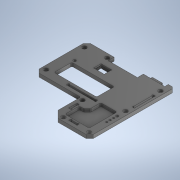
# Autodesk Inventor part: Cockpit_side_frame
Saved by Autodesk Inventor 2022.3 (Build 263350000, 350)
## iProperties
Part Number: Cockpit_side_frame
Material: アセタール樹脂、黒
Document SubType Name: Modeling
Designer: Masato Kubotera
Density: 1.425 g/cm^3
Appearance: 滑らか - 黒
Description: POM T5
Mass: 49.7941 g
Surface Area: 232.095 cm^2
Volume: 34.9432 cm^3
Author: Masato Kubotera
Autodesk Inventor part; units mm, degrees
ref_plane "YZ Plane" through (0, 0, 0) normal (1, 0, 0) x (0, 1, 0)
ref_plane "XZ Plane" through (0, 0, 0) normal (0, 1, 0) x (-1, 0, 0)
ref_plane "XY Plane" through (0, 0, 0) normal (0, 0, 1) x (1, 0, 0)
derived "Trunk_basis.ipt"
sketch "スケッチ1" plane through (0, 0, 0) normal (0, 1, 0) x (-1, 0, 0)
  line L0 (0, 22) -> (0, -142.9) construction
  circle A0 centre (5, 0) radius 10.5 construction
  line L1 (-7, 16) -> (36, 16) construction
  line L2 (36, 16) -> (36, -16) construction
  line L3 (36, -16) -> (-7, -16) construction
  line L4 (-7, -16) -> (-7, 16) construction
  line L5 (-7, 16) -> (36, -16) construction
  line L6 (36, 16) -> (-7, -16) construction
  line L7 (33, 13.5) -> (6, 13.5) construction
  line L8 (6, 13.5) -> (6, -13.5) construction
  line L9 (6, -13.5) -> (33, -13.5) construction
  line L10 (33, -13.5) -> (33, 13.5) construction
  line L11 (33, 13.5) -> (6, -13.5) construction
  line L12 (6, 13.5) -> (33, -13.5) construction
  line L13 (-7, 0) -> (36, 0) construction
  arc A1 (5, 16) -> (-7, 10.583) centre (5, 0) ccw construction
  line L14 (43.75, -16.25) -> (5, -16.25)
  line L15 (5, 16.25) -> (43.75, 16.25)
  line L16 (44.75, 15.25) -> (44.75, -15.25)
  arc A2 (5, 16.25) -> (-6.7376, 11.2379) centre (5, 0) ccw
  arc A3 (-6.7376, 11.2379) -> (-7.25, 9.9174) centre (-6.2711, 10.2972) ccw
  circle A4 centre (6, 13.5) radius 1.35
  line L17 (19.5, 13.5) -> (19.5, -13.5) construction
  circle A5 centre (33, 13.5) radius 1.35
  line L18 (-15, 22) -> (-20, 17)
  line L19 (-20, 17) -> (-20, -19)
  line L20 (-20, -19) -> (-28.5, -27.5)
  line L21 (-28.5, -27.5) -> (-28.5, -103)
  line L22 (57.5, -22.5) -> (57.5, 17)
  line L23 (57.5, 17) -> (52.5, 22)
  line L24 (52.5, 22) -> (-15, 22)
  line L25 (-35.5597, -116.5529) -> (-28.5, -142.9)
  line L26 (-16, -139) -> (-16, -94) construction
  line L27 (-7.5, -140.4849) -> (-7.5, -142.9)
  line L28 (-7.5, -142.9) -> (7.5, -142.9)
  line L29 (7.5, -140.4849) -> (7.5, -142.9)
  arc A6 (-7.5, -140.4849) -> (-8.9849, -139) centre (-8.2425, -139.7425) ccw
  line L30 (-17.5, -138.9955) -> (-17.5, -133) construction
  line L31 (-19, -133) -> (-16, -133) construction
  line L32 (-19, -133) -> (-19, -139) construction
  line L33 (-16, -133) -> (-16, -139) construction
  line L34 (-15, 22) -> (-10, 22) construction
  line L35 (-10, 22) -> (-10, -22) construction
  line L36 (-10, -22) -> (-15, -22) construction
  line L37 (-15, -22) -> (-15, 22) construction
  line L38 (-15, 22) -> (-10, -22) construction
  line L39 (-10, 22) -> (-15, -22) construction
  line L40 (-12.5, 22) -> (-12.5, -22) construction
  line L41 (-10, 0) -> (-15, 0) construction
  circle A7 centre (-12.5, 17.75) radius 1.6
  line L42 (-15, 10) -> (-12.5, 10) construction
  line L43 (-12.5, 10) -> (-12.5, -10) construction
  line L44 (-12.5, -10) -> (-15, -10) construction
  line L45 (-15, -10) -> (-15, 10) construction
  line L46 (-15, 10) -> (-12.5, -10) construction
  line L47 (-12.5, 10) -> (-15, -10) construction
  line L48 (-12.25, 10.25) -> (-15.25, 10.25)
  line L49 (-15.25, 8.15) -> (-15.25, -8.15)
  line L50 (-15.25, -10.25) -> (-12.25, -10.25)
  line L51 (-12.25, -8.15) -> (-12.25, 8.15)
  line L52 (-12.25, 10.25) -> (-15.25, -10.25) construction
  line L53 (-15.25, 10.25) -> (-12.25, -10.25) construction
  arc A8 (-15.25, 10.25) -> (-15.25, 8.15) centre (-15.25, 9.2) ccw
  line L54 (-13.75, 10) -> (-13.75, -10) construction
  arc A9 (-12.25, 8.15) -> (-12.25, 10.25) centre (-12.25, 9.2) ccw
  circle A10 centre (-12.5, -17.75) radius 1.6
  arc A11 (-15.25, -8.15) -> (-15.25, -10.25) centre (-15.25, -9.2) ccw
  arc A12 (-12.25, -10.25) -> (-12.25, -8.15) centre (-12.25, -9.2) ccw
  line L55 (36, 14.4) -> (44.5, 14.4) construction
  line L56 (44.5, 14.4) -> (44.5, -14.4) construction
  line L57 (36, -14.4) -> (44.5, -14.4) construction
  line L58 (49.95, 7.95) -> (49.95, -7.95)
  line L59 (52.5, 0) -> (47.5, 0) construction
  line L60 (47.5, 22) -> (52.5, 22) construction
  line L61 (52.55, -7.95) -> (52.55, 7.95)
  line L62 (51.25, 10) -> (51.25, -10) construction
  line L63 (52.5, 10) -> (50, -10) construction
  line L64 (52.5, -10) -> (50, -10) construction
  line L65 (52.5, 10) -> (52.5, -10) construction
  line L66 (50, 10) -> (52.5, -10) construction
  line L67 (49.95, -10.05) -> (52.55, -10.05)
  line L68 (49.95, 10.05) -> (52.55, -10.05) construction
  line L69 (52.55, 10.05) -> (49.95, -10.05) construction
  line L70 (52.5, -22) -> (47.5, -22) construction
  line L71 (47.5, 22) -> (52.5, -22) construction
  line L72 (52.5, 22) -> (52.5, -22) construction
  line L73 (52.5, 22) -> (47.5, -22) construction
  line L74 (50, 22) -> (50, -22) construction
  line L75 (47.5, -22) -> (47.5, 22) construction
  circle A13 centre (50, -17.75) radius 1.6
  arc A14 (52.55, -10.05) -> (52.55, -7.95) centre (52.55, -9) ccw
  line L76 (50, -10) -> (50, 10) construction
  arc A15 (49.95, -7.95) -> (49.95, -10.05) centre (49.95, -9) ccw
  arc A16 (49.95, 10.05) -> (49.95, 7.95) centre (49.95, 9) ccw
  arc A17 (52.55, 7.95) -> (52.55, 10.05) centre (52.55, 9) ccw
  line L77 (50, 10) -> (52.5, 10) construction
  line L78 (52.55, 10.05) -> (49.95, 10.05)
  circle A18 centre (50, 17.75) radius 1.6
  circle A19 centre (5, 0) radius 16 construction
  arc A20 (-6.7376, -11.2379) -> (5, -16.25) centre (5, 0) ccw
  arc A21 (-7.25, -9.9174) -> (-6.7376, -11.2379) centre (-6.2711, -10.2972) ccw
  line L79 (-7.25, -9.9174) -> (-7.25, 9.9174)
  line L80 (17.5, -138.9955) -> (17.5, -133) construction
  line L81 (19, -133) -> (19, -139) construction
  line L82 (16, -133) -> (16, -139) construction
  line L83 (19, -133) -> (16, -133) construction
  circle A22 centre (6, -13.5) radius 1.35
  circle A23 centre (33, -13.5) radius 1.35
  line L84 (-25.5, -142.9) -> (-7.5, -142.9) construction
  line L85 (25.5, -142.9) -> (7.5, -142.9) construction
  line L86 (-23.5, -22.5) -> (57.5, -22.5) construction
  line L87 (57.5, -22.5) -> (57.5, -103)
  circle A24 centre (-13.5, -55) radius 1.75
  line L88 (-11.5, -59) -> (45.5, -59)
  line L89 (47.5, -61) -> (47.5, -82.5)
  line L90 (45.5, -84.5) -> (-11.5, -84.5)
  line L91 (-13.5, -82.5) -> (-13.5, -61)
  line L92 (-13.5, -59) -> (47.5, -84.5) construction
  line L93 (47.5, -59) -> (-13.5, -84.5) construction
  line L94 (-11.5, -27.5) -> (45.5, -27.5)
  line L95 (47.5, -29.5) -> (47.5, -49)
  line L96 (45.5, -51) -> (-11.5, -51)
  line L97 (-13.5, -49) -> (-13.5, -29.5)
  line L98 (-13.5, -27.5) -> (47.5, -51) construction
  line L99 (47.5, -27.5) -> (-13.5, -51) construction
  line L100 (-23.5, -108) -> (-28.5, -103)
  circle A25 centre (-20.5415, -102) radius 1.6
  line L101 (-25.7227, -96) -> (25.7227, -96)
  line L102 (25.7227, -96) -> (34.9603, -112)
  line L103 (35.5597, -116.5529) -> (28.5, -142.9)
  line L104 (-25.7227, -96) -> (-34.9603, -112)
  line L105 (57.5, -103) -> (52.5, -108)
  arc A26 (-11.5, -27.5) -> (-13.5, -29.5) centre (-11.5, -29.5) ccw
  arc A27 (-13.5, -49) -> (-11.5, -51) centre (-11.5, -49) ccw
  arc A28 (45.5, -51) -> (47.5, -49) centre (45.5, -49) ccw
  arc A29 (47.5, -29.5) -> (45.5, -27.5) centre (45.5, -29.5) ccw
  arc A30 (-11.5, -59) -> (-13.5, -61) centre (-11.5, -61) ccw
  arc A31 (-13.5, -82.5) -> (-11.5, -84.5) centre (-11.5, -82.5) ccw
  arc A32 (45.5, -84.5) -> (47.5, -82.5) centre (45.5, -82.5) ccw
  arc A33 (47.5, -61) -> (45.5, -59) centre (45.5, -61) ccw
  line L106 (-23.5, -108) -> (52.5, -108)
  line L107 (-25.5, -139) -> (-25.5, -142.9)
  line L108 (-25.5, -142.9) -> (-28.5, -142.9)
  line L109 (-17.9813, -99.3843) -> (-16.9961, -101.0907)
  line L110 (-16.9961, -102.9093) -> (-17.9813, -104.6157)
  line L111 (-19.5563, -105.525) -> (-21.5266, -105.525)
  line L112 (-23.1016, -104.6157) -> (-24.0868, -102.9093)
  line L113 (-24.0868, -101.0907) -> (-23.1016, -99.3843)
  line L114 (-21.5266, -98.475) -> (-19.5563, -98.475)
  line L115 (-16, -94) -> (16, -94) construction
  arc A34 (-24.0868, -101.0907) -> (-24.0868, -102.9093) centre (-23.5618, -102) ccw
  arc A35 (-23.1016, -104.6157) -> (-21.5266, -105.525) centre (-22.0516, -104.6157) ccw
  arc A36 (-19.5563, -105.525) -> (-17.9813, -104.6157) centre (-19.0313, -104.6157) ccw
  arc A37 (-16.9961, -102.9093) -> (-16.9961, -101.0907) centre (-17.5211, -102) ccw
  arc A38 (-17.9813, -99.3843) -> (-19.5563, -98.475) centre (-19.0313, -99.3843) ccw
  arc A39 (-21.5266, -98.475) -> (-23.1016, -99.3843) centre (-22.0516, -99.3843) ccw
  line L116 (16, -139) -> (16, -94) construction
  line L117 (16, -94) -> (-16, -94) construction
  line L118 (-25.5, -139) -> (-8.9849, -139)
  line L119 (25.5, -142.9) -> (28.5, -142.9)
  arc A40 (8.9849, -139) -> (7.5, -140.4849) centre (8.2425, -139.7425) ccw
  circle A41 centre (29.7641, -115) radius 1.25
  line L120 (33.4891, -124.2803) -> (21.898, -121.1745) construction
  line L121 (29.7641, -115) -> (25.623, -130.4548) construction
  circle A42 centre (29.7641, -115) radius 6 construction
  circle A43 centre (-20.5415, -102) radius 6 construction
  line L122 (1.9319, -109.4824) -> (7.5588, -130.4824)
  line L123 (5.6269, -133) -> (-5.6269, -133)
  line L124 (5.3151, -110.5176) -> (10.942, -131.5176)
  line L125 (12.8739, -133) -> (17.1947, -133)
  line L126 (19.1266, -131.5176) -> (24.7535, -110.5176)
  line L127 (22.8217, -108) -> (7.2469, -108)
  circle A44 centre (25.623, -130.4548) radius 1.25
  circle A45 centre (25.623, -130.4548) radius 6 construction
  line L128 (-1.9319, -109.4824) -> (-7.5588, -130.4824)
  arc A46 (1.9319, -109.4824) -> (-1.9319, -109.4824) centre (0, -110) ccw
  arc A47 (-7.5588, -130.4824) -> (-5.6269, -133) centre (-5.6269, -131) ccw
  arc A48 (5.6269, -133) -> (7.5588, -130.4824) centre (5.6269, -131) ccw
  arc A49 (7.2469, -108) -> (5.3151, -110.5176) centre (7.2469, -110) ccw
  arc A50 (24.7535, -110.5176) -> (22.8217, -108) centre (22.8217, -110) ccw
  arc A51 (17.1947, -133) -> (19.1266, -131.5176) centre (17.1947, -131) ccw
  arc A52 (10.942, -131.5176) -> (12.8739, -133) centre (12.8739, -131) ccw
  arc A53 (-5.3151, -110.5176) -> (-7.2469, -108) centre (-7.2469, -110) ccw
  line L129 (-22.8217, -108) -> (-7.2469, -108)
  line L130 (-5.3151, -110.5176) -> (-10.942, -131.5176)
  arc A54 (-22.8217, -108) -> (-24.7535, -110.5176) centre (-22.8217, -110) ccw
  line L131 (-19.1266, -131.5176) -> (-24.7535, -110.5176)
  arc A55 (-19.1266, -131.5176) -> (-17.1947, -133) centre (-17.1947, -131) ccw
  line L132 (-12.8739, -133) -> (-17.1947, -133)
  arc A56 (-12.8739, -133) -> (-10.942, -131.5176) centre (-12.8739, -131) ccw
  circle A57 centre (-29.7641, -115) radius 1.25
  circle A58 centre (-25.623, -130.4548) radius 1.25
  arc A59 (35.5597, -116.5529) -> (34.9603, -112) centre (29.7641, -115) ccw
  arc A60 (-34.9603, -112) -> (-35.5597, -116.5529) centre (-29.7641, -115) ccw
  arc A61 (-24.0151, -139) -> (-25.5, -140.4849) centre (-24.7575, -139.7425) ccw
  line L133 (25.5, -139) -> (25.5, -142.9)
  arc A62 (25.5, -140.4849) -> (24.0151, -139) centre (24.7575, -139.7425) ccw
  line L134 (25.5, -139) -> (8.9849, -139)
  line L135 (21.5266, -98.475) -> (19.5563, -98.475)
  line L136 (16.9961, -102.9093) -> (17.9813, -104.6157)
  arc A63 (21.5266, -105.525) -> (23.1016, -104.6157) centre (22.0516, -104.6157) ccw
  circle A64 centre (20.5415, -102) radius 1.6
  line L137 (24.0868, -101.0907) -> (23.1016, -99.3843)
  arc A65 (24.0868, -102.9093) -> (24.0868, -101.0907) centre (23.5618, -102) ccw
  line L138 (23.1016, -104.6157) -> (24.0868, -102.9093)
  arc A66 (23.1016, -99.3843) -> (21.5266, -98.475) centre (22.0516, -99.3843) ccw
  line L139 (19.5563, -105.525) -> (21.5266, -105.525)
  arc A67 (19.5563, -98.475) -> (17.9813, -99.3843) centre (19.0313, -99.3843) ccw
  arc A68 (17.9813, -104.6157) -> (19.5563, -105.525) centre (19.0313, -104.6157) ccw
  line L140 (17.9813, -99.3843) -> (16.9961, -101.0907)
  arc A69 (16.9961, -101.0907) -> (16.9961, -102.9093) centre (17.5211, -102) ccw
  line L141 (16, -139) -> (16, -94) construction
  circle A70 centre (20.5415, -102) radius 6 construction
  arc A71 (29.5045, -117.5445) -> (31.2612, -117.0738) centre (30.247, -116.802) ccw construction
  line L142 (31.8379, -116.4971) -> (31.2612, -117.0738) construction
  line L143 (29.5045, -117.5445) -> (28.7167, -117.3334) construction
  arc A72 (27.4307, -116.0474) -> (28.7167, -117.3334) centre (28.4449, -116.3192) ccw construction
  line L144 (27.4307, -116.0474) -> (27.2196, -115.2596) construction
  line L145 (27.6903, -113.5029) -> (28.267, -112.9262) construction
  arc A73 (30.0237, -112.4555) -> (28.267, -112.9262) centre (29.2813, -113.198) ccw construction
  arc A74 (27.6903, -113.5029) -> (27.2196, -115.2596) centre (27.9621, -114.5171) ccw construction
  line L146 (30.0237, -112.4555) -> (30.8116, -112.6666) construction
  arc A75 (31.8379, -116.4971) -> (32.3086, -114.7404) centre (31.5662, -115.4829) ccw construction
  arc A76 (32.0975, -113.9526) -> (30.8116, -112.6666) centre (31.0833, -113.6808) ccw construction
  line L147 (32.0975, -113.9526) -> (32.3086, -114.7404) construction
  line L148 (-20.5415, -102) -> (20.5415, -102) construction
  circle A77 centre (0, -102) radius 1.6
  line L149 (0.4078, -104.525) -> (-0.4078, -104.525)
  arc A78 (-0.4078, -99.475) -> (-1.9828, -100.3843) centre (-0.9328, -100.3843) ccw
  arc A79 (0.4078, -104.525) -> (1.9828, -103.6157) centre (0.9328, -103.6157) ccw
  line L150 (2.3906, -102.9093) -> (1.9828, -103.6157)
  line L151 (-0.4078, -99.475) -> (0.4078, -99.475)
  arc A80 (1.9828, -100.3843) -> (0.4078, -99.475) centre (0.9328, -100.3843) ccw
  line L152 (1.9828, -100.3843) -> (2.3906, -101.0907)
  arc A81 (2.3906, -102.9093) -> (2.3906, -101.0907) centre (1.8656, -102) ccw
  line L153 (-2.3906, -101.0907) -> (-1.9828, -100.3843)
  arc A82 (-2.3906, -101.0907) -> (-2.3906, -102.9093) centre (-1.8656, -102) ccw
  line L154 (-1.9828, -103.6157) -> (-2.3906, -102.9093)
  arc A83 (-1.9828, -103.6157) -> (-0.4078, -104.525) centre (-0.9328, -103.6157) ccw
  circle A84 centre (0, -102) radius 1.25
  arc A85 (44.75, 15.25) -> (43.75, 16.25) centre (43.75, 15.25) ccw
  arc A86 (43.75, -16.25) -> (44.75, -15.25) centre (43.75, -15.25) ccw
  circle A87 centre (-22.75, -31.75) radius 3
  circle A88 centre (-22.75, -86.75) radius 3
  line L155 (-23.5, -96) -> (-28.5, -91) construction
  line L156 (-26, -93.5) -> (-22.75, -93.5) construction
  line L157 (-26, -25) -> (-22.75, -25) construction
  line L158 (-26, -25) -> (-26, -93.5) construction
  line L159 (-22.75, -25) -> (-22.75, -93.5) construction
  line L160 (-22.75, -59.25) -> (-28.5, -59.25) construction
  point P0 (0, 0)
  point P1 (14.5, 0)
  point P2 (19.5, 0)
  point P3 (44.75, 16.25)
  point P4 (-7.25, 10.6771)
  point P5 (19.5, 0)
  point P6 (-12.5, 0)
  point P7 (-13.75, 0)
  point P8 (44.75, 14.4)
  point P9 (44.75, -14.4)
  point P10 (51.25, 0)
  point P11 (50, 0)
  point P12 (44.75, -16.25)
  point P13 (17, -71.75)
  point P14 (17, -39.25)
  point P15 (-18.5063, -98.475)
  point P16 (-16.4711, -102)
  point P17 (-18.5063, -105.525)
  point P18 (-22.5766, -105.525)
  point P19 (-22.5766, -98.475)
  point P20 (-24.6118, -102)
  point P21 (-22.5766, -105.525)
  point P22 (-18.5063, -105.525)
  point P23 (-16.4711, -102)
  point P24 (-18.5063, -98.475)
  point P25 (-22.5766, -98.475)
  point P26 (27.6936, -122.7274)
  point P27 (0, -102.2726)
  point P28 (0, -133)
  point P29 (-7.5, -139)
  point P30 (-22.5766, -98.475)
  point P31 (18.5063, -98.475)
  point P32 (18.5063, -98.475)
  point P33 (22.5766, -105.525)
  point P34 (22.5766, -105.525)
  point P35 (24.6118, -102)
  point P36 (22.5766, -98.475)
  point P37 (22.5766, -98.475)
  point P38 (22.5766, -98.475)
  point P39 (18.5063, -105.525)
  point P40 (16.4711, -102)
  point P41 (16.4711, -102)
  point P42 (18.5063, -105.525)
  point P43 (29.7641, -115)
  point P44 (29.7641, -115)
  point P45 (30.5187, -117.8163)
  point P46 (30.5187, -117.8163)
  point P47 (27.7025, -117.0617)
  point P48 (27.7025, -117.0617)
  point P49 (31.8258, -112.9383)
  point P50 (26.9479, -114.2454)
  point P51 (29.0095, -112.1837)
  point P52 (29.0095, -112.1837)
  point P53 (31.8258, -112.9383)
  point P54 (29.0095, -112.1837)
  point P55 (32.5804, -115.7546)
  point P56 (-1.4578, -99.475)
  point P57 (-1.4578, -99.475)
  point P58 (-1.4578, -99.475)
  point P59 (1.4578, -104.525)
  point P60 (1.4578, -99.475)
  point P61 (1.4578, -99.475)
  point P62 (2.9156, -102)
  point P63 (-2.9156, -102)
  point P64 (-1.4578, -104.525)
  point P65 (-1.4578, -104.525)
sketch "スケッチ2" plane through (0, 0, 0) normal (0, 1, 0) x (-1, 0, 0)
  line L0 (-23.5, -22.5) -> (-28.5, -27.5)
  line L1 (-28.5, -27.5) -> (-28.5, -91)
  line L2 (-28.5, -91) -> (-23.5, -96)
  line L3 (-23.5, -96) -> (34.25, -96)
  line L4 (36.25, -98) -> (36.25, -128.5)
  line L5 (36.25, -128.5) -> (46.25, -138.5)
  line L6 (46.25, -138.5) -> (86.5, -138.5)
  line L7 (91.5, -133.5) -> (91.5, -20)
  line L8 (91.5, -20) -> (89, -17.5)
  line L9 (89, -17.5) -> (83.25, -17.5)
  line L10 (83.25, -17.5) -> (83.25, -21.0151)
  line L11 (81.7651, -22.5) -> (76.8599, -22.5)
  line L12 (75.375, -21.0151) -> (75.375, -17.5)
  line L13 (75.375, -17.5) -> (60.375, -17.5)
  line L14 (60.375, -17.5) -> (60.375, -21.0151)
  line L15 (58.8901, -22.5) -> (-23.5, -22.5)
  line L16 (-25.25, -25) -> (-20.25, -25) construction
  line L17 (-20.25, -25) -> (-20.25, -93.5) construction
  line L18 (-20.25, -93.5) -> (-25.25, -93.5) construction
  line L19 (-25.25, -93.5) -> (-25.25, -25) construction
  line L20 (-26, -25) -> (-25.25, -25) construction
  line L21 (-25.25, -93.5) -> (-26, -93.5) construction
  line L22 (-26, -93.5) -> (-26, -25) construction
  line L23 (-20.25, -93.5) -> (83.25, -93.5) construction
  line L24 (-20.25, -88.5) -> (83.25, -88.5) construction
  line L25 (83.25, -22.5) -> (83.25, -90) construction
  line L26 (83.25, -90) -> (88.25, -90) construction
  line L27 (88.25, -90) -> (88.25, -22.5) construction
  line L28 (83.25, -88.5) -> (83.25, -93.5) construction
  line L29 (83.25, -91) -> (88.25, -91) construction
  line L30 (88.25, -91) -> (88.25, -136) construction
  line L31 (83.25, -91) -> (83.25, -136) construction
  line L32 (83.25, -136) -> (88.25, -136) construction
  line L33 (38.75, -131) -> (38.75, -93.5) construction
  line L34 (43.75, -93.5) -> (43.75, -131) construction
  line L35 (38.75, -131) -> (43.75, -131) construction
  line L36 (41.25, -131) -> (41.25, -93.5) construction
  line L37 (43.75, -131) -> (81.25, -131) construction
  line L38 (81.25, -131) -> (81.25, -136) construction
  line L39 (81.25, -136) -> (43.75, -136) construction
  line L40 (43.75, -133.5) -> (81.25, -133.5) construction
  line L41 (85.75, -91) -> (85.75, -136) construction
  circle A0 centre (85.75, -133.5) radius 2.975
  arc A1 (83.25, -131) -> (88.25, -131) centre (85.75, -133.5) ccw construction
  line L42 (83.25, -91) -> (-20.25, -91) construction
  line L43 (41.25, -112.25) -> (43.75, -112.25) construction
  line L44 (62.5, -131) -> (62.5, -133.5) construction
  line L45 (41.2, -116.8151) -> (41.2, -107.6849)
  line L46 (43.8, -108.3) -> (43.8, -116.2)
  line L47 (43.8, -118.3) -> (41.2, -106.2) construction
  line L48 (41.2, -118.3) -> (43.8, -106.2) construction
  line L49 (58.55, -130.95) -> (66.45, -130.95)
  line L50 (67.0651, -133.55) -> (57.9349, -133.55)
  line L51 (56.45, -130.95) -> (68.55, -133.55) construction
  line L52 (68.55, -130.95) -> (56.45, -133.55) construction
  line L53 (41.25, -106.25) -> (43.75, -106.25) construction
  line L54 (41.25, -118.25) -> (43.75, -118.25) construction
  arc A2 (42.6849, -106.2) -> (41.2, -107.6849) centre (41.9425, -106.9425) ccw
  arc A3 (43.8, -108.3) -> (43.8, -106.2) centre (43.8, -107.25) ccw
  arc A4 (41.2, -116.8151) -> (42.6849, -118.3) centre (41.9425, -117.5575) ccw
  arc A5 (43.8, -118.3) -> (43.8, -116.2) centre (43.8, -117.25) ccw
  line L55 (56.5, -133.5) -> (56.5, -131) construction
  line L56 (68.5, -131) -> (68.5, -133.5) construction
  arc A6 (56.45, -132.0651) -> (57.9349, -133.55) centre (57.1925, -132.8075) ccw
  arc A7 (58.55, -130.95) -> (56.45, -130.95) centre (57.5, -130.95) ccw
  arc A8 (67.0651, -133.55) -> (68.55, -132.0651) centre (67.8075, -132.8075) ccw
  arc A9 (68.55, -130.95) -> (66.45, -130.95) centre (67.5, -130.95) ccw
  line L57 (56.45, -132.0651) -> (56.45, -130.95)
  line L58 (68.55, -130.95) -> (68.55, -132.0651)
  line L59 (42.6849, -106.2) -> (43.8, -106.2)
  line L60 (43.8, -118.3) -> (42.6849, -118.3)
  circle A10 centre (48.75, -133.5) radius 1.6
  line L61 (88.25, -22.5) -> (88.25, -17.5) construction
  line L62 (89, -17.5) -> (89, -90) construction
  line L63 (89, -90) -> (88.25, -90) construction
  line L64 (-13.5, -82.5) -> (-13.5, -61) projected
  arc A11 (-13.5, -82.5) -> (-11.5, -84.5) centre (-11.5, -82.5) ccw projected
  line L65 (45.5, -84.5) -> (-11.5, -84.5) projected
  arc A12 (45.5, -84.5) -> (47.5, -82.5) centre (45.5, -82.5) ccw projected
  line L66 (47.5, -61) -> (47.5, -82.5) projected
  arc A13 (47.5, -61) -> (45.5, -59) centre (45.5, -61) ccw projected
  line L67 (-11.5, -59) -> (45.5, -59) projected
  arc A14 (-11.5, -59) -> (-13.5, -61) centre (-11.5, -61) ccw projected
  line L68 (31.5, -88.5) -> (31.5, -91) construction
  line L69 (85.75, -22.5) -> (85.75, -90) construction
  circle A15 centre (85.75, -31.25) radius 1.6
  circle A16 centre (85.75, -31.25) radius 3
  circle A17 centre (85.75, -81.25) radius 1.6
  circle A18 centre (85.75, -81.25) radius 3
  line L70 (88.25, -22.5) -> (83.25, -22.5) construction
  arc A19 (88.25, -91) -> (83.25, -91) centre (85.75, -133.5) ccw construction
  circle A20 centre (48.75, -133.5) radius 3
  circle A21 centre (41.25, -98.5) radius 1.6
  circle A22 centre (41.25, -98.5) radius 3
  line L71 (10.55, -88.5) -> (10.55, -91) construction
  line L72 (52.45, -88.5) -> (52.45, -91) construction
  line L73 (51.0151, -91.05) -> (11.9849, -91.05)
  line L74 (10.5, -89.5651) -> (10.5, -88.45)
  line L75 (12.6, -88.45) -> (50.4, -88.45)
  line L76 (52.5, -88.45) -> (52.5, -89.5651)
  line L77 (52.5, -91.05) -> (10.5, -88.45) construction
  line L78 (10.5, -91.05) -> (52.5, -88.45) construction
  arc A23 (12.6, -88.45) -> (10.5, -88.45) centre (11.55, -88.45) ccw
  arc A24 (10.5, -89.5651) -> (11.9849, -91.05) centre (11.2425, -90.3075) ccw
  arc A25 (52.5, -88.45) -> (50.4, -88.45) centre (51.45, -88.45) ccw
  arc A26 (51.0151, -91.05) -> (52.5, -89.5651) centre (51.7575, -90.3075) ccw
  line L79 (-20.25, -31) -> (83.25, -31) construction
  line L80 (83.25, -26) -> (-20.25, -26) construction
  line L81 (-20.25, -26) -> (-20.25, -31) construction
  line L82 (-20.25, -28.5) -> (83.25, -28.5) construction
  line L83 (31.5, -31) -> (31.5, -26) construction
  line L84 (11.9849, -31.05) -> (51.0151, -31.05)
  arc A27 (10.5, -29.5651) -> (11.9849, -31.05) centre (11.2425, -30.3075) ccw
  arc A28 (51.0151, -31.05) -> (52.5, -29.5651) centre (51.7575, -30.3075) ccw
  line L85 (10.55, -31) -> (10.55, -26) construction
  line L86 (52.45, -26) -> (52.45, -31) construction
  circle A29 centre (6.5, -28.5) radius 1.6
  circle A30 centre (6.5, -28.5) radius 3
  line L87 (-26, -59.25) -> (-25.25, -59.25) construction
  line L88 (-22.75, -25) -> (-22.75, -93.5) construction
  arc A31 (58.8901, -22.5) -> (60.375, -21.0151) centre (59.6325, -21.7575) ccw
  arc A32 (75.375, -21.0151) -> (76.8599, -22.5) centre (76.1175, -21.7575) ccw
  line L89 (56.4375, -22.5) -> (56.4375, -17.5) construction
  line L90 (79.3125, -22.5) -> (79.3125, -17.5) construction
  circle A33 centre (-22.75, -31.75) radius 1.6
  circle A34 centre (-22.75, -31.75) radius 3
  circle A35 centre (-22.75, -86.75) radius 1.6
  circle A36 centre (-22.75, -86.75) radius 3
  line L91 (60.375, -22.5) -> (75.375, -22.5)
  line L92 (52.5, -17.5) -> (52.5, -22.5) construction
  circle A37 centre (85.75, -98.5) radius 1.475
  circle A38 centre (85.75, -103.5) radius 1.475
  circle A39 centre (85.75, -108.5) radius 1.475
  line L93 (59.5, -88.5) -> (78.75, -88.5)
  line L94 (80.75, -90.5) -> (80.75, -126.5)
  line L95 (78.75, -128.5) -> (48.25, -128.5)
  line L96 (46.25, -126.5) -> (46.25, -110)
  arc A40 (46.25, -126.5) -> (48.25, -128.5) centre (48.25, -126.5) ccw
  arc A41 (78.75, -128.5) -> (80.75, -126.5) centre (78.75, -126.5) ccw
  arc A42 (80.75, -90.5) -> (78.75, -88.5) centre (78.75, -90.5) ccw
  arc A43 (36.25, -98) -> (34.25, -96) centre (34.25, -98) ccw
  circle A44 centre (-13.5, -55) radius 1.75 projected
  circle A45 centre (-13.5, -55) radius 2
  line L97 (23.9, -49.9425) -> (10.1, -49.9425) construction
  line L98 (10.1, -49.9425) -> (10.1, -40.7425) construction
  line L99 (10.1, -40.7425) -> (23.9, -40.7425) construction
  line L100 (23.9, -40.7425) -> (23.9, -49.9425) construction
  line L101 (23.9, -49.9425) -> (10.1, -40.7425) construction
  line L102 (10.1, -49.9425) -> (23.9, -40.7425) construction
  line L103 (9.45, -40.0425) -> (24.55, -40.0425) construction
  line L104 (24.55, -40.0425) -> (24.55, -50.6425) construction
  line L105 (24.55, -50.6425) -> (9.45, -50.6425) construction
  line L106 (9.45, -50.6425) -> (9.45, -40.0425) construction
  line L107 (9.45, -40.0425) -> (24.55, -50.6425) construction
  line L108 (24.55, -40.0425) -> (9.45, -50.6425) construction
  line L109 (10.8849, -39.9925) -> (23.1151, -39.9925)
  line L110 (24.6, -41.4774) -> (24.6, -49.2075)
  line L111 (24.6, -50.6925) -> (9.4, -39.9925) construction
  line L112 (9.4, -50.6925) -> (24.6, -39.9925) construction
  line L113 (23.95, -49.9925) -> (10.05, -40.6925) construction
  line L114 (10.05, -49.9925) -> (23.95, -40.6925) construction
  arc A46 (10.8849, -39.9925) -> (9.4, -41.4774) centre (10.1425, -40.7349) ccw
  arc A47 (11.5349, -40.6925) -> (10.05, -42.1774) centre (10.7925, -41.4349) ccw
  line L115 (9.4, -45.3425) -> (24.6, -45.3425) construction
  line L116 (17, -39.9925) -> (17, -50.6925) construction
  arc A48 (24.6, -41.4774) -> (23.1151, -39.9925) centre (23.8575, -40.7349) ccw
  arc A49 (23.95, -42.1774) -> (22.4651, -40.6925) centre (23.2075, -41.4349) ccw
  arc A50 (9.4, -49.2075) -> (10.8849, -50.6925) centre (10.1425, -49.95) ccw
  arc A51 (10.05, -48.5075) -> (11.5349, -49.9925) centre (10.7925, -49.25) ccw
  arc A52 (23.1151, -50.6925) -> (24.6, -49.2075) centre (23.8575, -49.95) ccw
  arc A53 (22.4651, -49.9925) -> (23.95, -48.5075) centre (23.2075, -49.25) ccw
  line L117 (11.5349, -40.6925) -> (22.4651, -40.6925)
  line L118 (23.95, -42.1774) -> (23.95, -48.5075)
  line L119 (9.4, -49.2075) -> (9.4, -41.4774)
  line L120 (10.05, -48.5075) -> (10.05, -42.1774)
  line L121 (22.4651, -49.9925) -> (11.5349, -49.9925)
  line L122 (23.1151, -50.6925) -> (10.8849, -50.6925)
  line L123 (-13.5, -71.75) -> (47.5, -71.75) construction
  line L124 (85.75, -56.25) -> (88.25, -56.25) construction
  line L125 (85.7, -69.2) -> (85.7, -43.3)
  line L126 (88.3049, -71.3569) -> (85.7, -41.2) construction
  line L127 (85.7, -71.3) -> (88.3, -41.2) construction
  arc A54 (85.7, -41.2) -> (85.7, -43.3) centre (85.7, -42.25) ccw
  arc A55 (88.3, -42.6849) -> (86.8151, -41.2) centre (87.5575, -41.9425) ccw
  arc A56 (85.7, -69.2) -> (85.7, -71.3) centre (85.7, -70.25) ccw
  arc A57 (86.8151, -71.3) -> (88.3, -69.8151) centre (87.5575, -70.5575) ccw
  line L128 (85.75, -41.25) -> (88.25, -41.25) construction
  line L129 (85.75, -71.25) -> (88.25, -71.25) construction
  line L130 (88.3, -42.6849) -> (88.3, -69.8151)
  line L131 (88.3, -66.8652) -> (88.3, -69.8151)
  line L132 (86.8151, -71.3) -> (85.7, -71.3)
  line L133 (85.7, -41.2) -> (86.8151, -41.2)
  line L134 (86.5, -138.5) -> (91.5, -133.5)
  arc A58 (81.7651, -22.5) -> (83.25, -21.0151) centre (82.5075, -21.7575) ccw
  circle A59 centre (85.75, -93.5) radius 2
  circle A60 centre (85.75, -93.5) radius 4 construction
  arc A61 (-13.5, -49) -> (-11.5, -51) centre (-11.5, -49) ccw construction
  line L135 (45.5, -51) -> (-11.5, -51) construction
  arc A62 (45.5, -51) -> (47.5, -49) centre (45.5, -49) ccw construction
  line L136 (10.5, -29.5651) -> (10.5, -22.5)
  line L137 (52.5, -29.5651) -> (52.5, -22.5)
  line L138 (67.875, -17.5) -> (67.875, -22.5) construction
  line L139 (52.5, -17.5) -> (83.25, -17.5) construction
  line L140 (43.75, -131) -> (43.75, -136) construction
  line L141 (57.5, -22.5) -> (57.5, -103) construction
  line L142 (57.5, -103) -> (52.5, -108) construction
  line L143 (-23.5, -108) -> (52.5, -108) construction
  line L144 (57.5, -90.5) -> (57.5, -102.1716)
  line L145 (56.9142, -103.5858) -> (53.0858, -107.4142)
  line L146 (51.6716, -108) -> (48.25, -108)
  arc A63 (59.5, -88.5) -> (57.5, -90.5) centre (59.5, -90.5) ccw
  arc A64 (56.9142, -103.5858) -> (57.5, -102.1716) centre (55.5, -102.1716) ccw
  arc A65 (51.6716, -108) -> (53.0858, -107.4142) centre (51.6716, -106) ccw
  arc A66 (48.25, -108) -> (46.25, -110) centre (48.25, -110) ccw
  point P0 (0, 0)
  point P1 (-25.7227, -96)
  point P2 (-23.5, -22.5)
  point P3 (42.5, -112.25)
  point P4 (62.5, -132.25)
  point P5 (31.5, -89.75)
  point P6 (31.5, -28.5)
  point P7 (52.5, -22)
  point P8 (46.25, -108)
  point P9 (57.5, -88.5)
  point P10 (17, -45.3425)
  point P11 (17, -45.3425)
  point P12 (87, -56.25)
  point P13 (17, -51)
  point P14 (10.5, -31.05)
  dimension "d1" = 120
  dimension "d2" = 5
  dimension "d3" = 0.75
  dimension "d9" = 15
  dimension "d11" = 5
  dimension "d12" = 68.5
  dimension "d13" = 5
  dimension "d15" = 5
  dimension "d16" = 2.5
  dimension "d19" = 5.95
  dimension "d20" = 0.9645
  dimension "d21" = 37.5
  dimension "d22" = 39.5
  dimension "d24" = 2.5
  dimension "d25" = 5
  dimension "d26" = 12
  dimension "d28" = 0.05
  dimension "d31" = 12
  dimension "d32" = 0.05
  dimension "d36" = 0.05
  dimension "d37" = 0.05
  dimension "d39" = 0.75
  dimension "d40" = 5
  dimension "d43" = 50
  dimension "d44" = 0.9265
  dimension "d48" = 27.5
  dimension "d49" = 41.9
  dimension "d52" = 0.05
  dimension "d53" = 0.05
  dimension "d54" = 5
  dimension "d55" = 3.5
  dimension "d57" = 41.9
  dimension "d62" = 72.5
  dimension "d68" = 1.05
  dimension "d71" = 39
  dimension "d82" = 1
  dimension "d83" = 3.2
  dimension "d84" = 6
  dimension "d85" = 55
  dimension "d86" = 2.95
  dimension "d87" = 7.5
  dimension "d90" = 5
  dimension "d96" = 2.5
  dimension "d97" = 2.5
  dimension "d98" = 2
  dimension "d101" = 4
  dimension "d104" = 13.8
  dimension "d105" = 9.2
  dimension "d106" = 15.1
  dimension "d107" = 10.6
  dimension "d108" = 0.05
  dimension "d112" = 1.05
  dimension "d113" = 1.05
  dimension "d114" = 0.05
  dimension "d115" = 0.05
  dimension "d116" = 0.05
  dimension "d118" = 1.05
  dimension "d119" = 1.05
  dimension "d120" = 30
  dimension "d122" = 0.05
  dimension "d127" = 0.05
  dimension "d128" = 5
  dimension "d129" = 5
  dimension "d130" = 2.5
  constraints: 277 end point, 100 point on line, 98 point on circle, 60 centre point, 59 midpoint, 47 perpendicular, 42 symmetric about line, 30 parallel, 22 equal radius, 17 tangent, 14 horizontal, 12 coincident, 10 vertical, 9 collinear, 39 other
  measures "d1" distance between parallel lines of L1 L7
  measures "d2" distance of L16.start L16.end
  measures "d3" distance of L20.start L20.end
  measures "d9" distance of L12.end L13.end
  measures "d11" horizontal distance of L2.end L1.end
  measures "d12" distance of L21.end L20.start
  measures "d13" distance of L33.end L34.start
  measures "d15" distance of L31.end L30.end
  measures "d16" distance between parallel lines of L6 L39
  measures "d19" diameter of A0
  measures "d20" distance edge to line of A1 L38
  measures "d21" distance of L34.start L34.end
  measures "d22" distance between parallel lines of L31 L34
  measures "d24" distance between parallel lines of L3 L23
  measures "d25" distance of L24.end L23.end
  measures "d26" distance of L54.end L53.end
  measures "d28" distance between parallel lines of L46 L34
  measures "d31" distance between parallel lines of L56 L55
  measures "d32" distance between parallel lines of L49 L37
  measures "d36" distance between parallel lines of L57 L55
  measures "d37" distance between parallel lines of L59 L53
  measures "d39" distance of L62.end L26.end
  measures "d40" distance of L27.end L61.end
  measures "d43" distance of A18.centre A15.centre
  measures "d44" distance edge to line of A19 L26
  measures "d48" diameter of A22.centre L43
  measures "d49" distance between parallel lines of L72 L71
  measures "d52" distance between parallel lines of L24 L75
  measures "d53" distance between parallel lines of L71 L74
  measures "d54" distance between parallel lines of L79 L80
  measures "d55" distance between parallel lines of L80 L70
  measures "d57" distance between parallel lines of L85 L86
  measures "d62" distance of L62.end L8.end
  measures "d68" radius of A31
  measures "d71" distance from line of L7 point (52.5, -22)
  measures "d82" distance between parallel lines of L29 L26
  measures "d83" diameter of A33
  measures "d84" diameter of A34
  measures "d85" distance of A35.centre A33.centre
  measures "d86" diameter of A37
  measures "d87" distance of A37.centre L41.start
  measures "d90" distance of A37.centre A38.centre
  measures "d96" distance between parallel lines of L34 L96
  measures "d97" distance between parallel lines of L37 L95
  measures "d98" radius of A43
  measures "d101" diameter of A45
  measures "d104" distance of L98.end L99.end
  measures "d105" distance of L97.end L98.end
  measures "d106" distance of L104.end L105.end
  measures "d107" distance of L103.end L104.end
  measures "d108" distance between parallel lines of L109 L103
  measures "d112" radius of A46
  measures "d113" radius of A47
  measures "d114" distance between parallel lines of L117 L99
  measures "d115" distance between parallel lines of L119 L106
  measures "d116" distance between parallel lines of L120 L98
  measures "d118" radius of A55
  measures "d119" radius of A54
  measures "d120" distance between parallel lines of L129 L128
  measures "d122" distance between parallel lines of L125 L69
  measures "d127" distance between parallel lines of L133 L128
  measures "d128" distance from line of L6.end L7
  measures "d129" horizontal distance of L6.end L7.start
  measures "d130" horizontal distance of L7.end L8.end
extrude "押し出し1" add sketch "スケッチ2" along normal blind 5 contours L15 L136 A27 L84 A28 L137 A31 L91 A32 L11 A58 L10 L9 L8 L7 L134 L6 L5 L4 A43 L3 L2 L1 L0
extrude "押し出し2" add sketch "スケッチ2" along normal blind 2.5 contours A31 L14 L13 L12 A32 L91
extrude "押し出し3" add sketch "スケッチ2" along normal blind 1.9 contours A16 | A18 | A20 | A22 | A30 | A34 | A36
extrude "押し出し4" add sketch "スケッチ2" along normal blind 0.5 contours L93 A42 L94 A41 L95 A40 L96 A66 L146 A65 L145 A64 L144 A63
extrude "押し出し5" add sketch "スケッチ2" along normal blind 3 contours L109 A48 L110 A52 L122 A50 L119 A46
sketch "スケッチ3" plane through (-83.25, 0, -22.5) normal (0, 0, 1) x (1, 0, 0)
  line L0 (1.4849, 5) -> (6.3901, 5) projected
  line L1 (3.9375, 5) -> (3.9375, 0)
  line L2 (24.3599, 5) -> (106.75, 5) projected
  line L3 (1.4849, 0) -> (6.3901, 0) projected
  point P0 (83.25, 0)
  point P1 (26.8125, 0)
  point P2 (0, 0)
  point P3 (3.9375, 2.5)
  constraints: 2 end point, 2 midpoint, 1 vertical
hole "穴1" at (-79.3125, 2.5, -22.5) direction (0, 0, -1) diameter 3.4587 depth 4 thread size "M4x0.5" class "6H" standard "ISO Metric profile"
chamfer "面取り1" distance 0.5 angle 45 2 edges at (-75.375, 1.25, -17.5) (-60.375, 1.25, -17.5)
